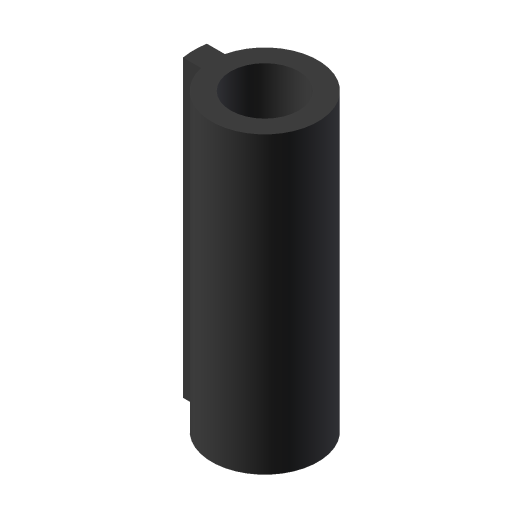
# Autodesk Inventor part: Servo Adapter
Saved by Autodesk Inventor 2023.4 (Build 274418000, 418)
## iProperties
Created: 2024-02-27
Part Number: Servo Adapter
Material: Generic
Document SubType Name: Modeling
Designer: josep
Density: 1 g/cm^3
Appearance: Default
Author: josep
Autodesk Inventor part; units mm, degrees
ref_plane "YZ Plane" through (0, 0, 0) normal (1, 0, 0) x (0, 1, 0)
ref_plane "XZ Plane" through (0, 0, 0) normal (0, 1, 0) x (-1, 0, 0)
ref_plane "XY Plane" through (0, 0, 0) normal (0, 0, 1) x (1, 0, 0)
sketch "Sketch1" plane through (0, 0, 0) normal (0, 1, 0) x (-1, 0, 0)
  circle A0 centre (0, 0) radius 4.5
  circle A1 centre (0, 0) radius 2.9
  circle A2 centre (0, 0) radius 6
  line L0 (4.3875, -1) -> (5.9161, -1)
  line L1 (4.3875, 1) -> (5.9161, 1)
  dimension "d0" = 0
  dimension "d1" = 0
  dimension "d2" = 9
  dimension "d3" = 5.8
  dimension "d4" = 12
  dimension "d5" = 1
  dimension "d6" = 1
  constraints: 4 end point, 4 point on circle, 3 centre point, 2 coincident, 1 horizontal, 1 parallel
  measures "d0" distance of point (0, 0) A0.centre
  measures "d1" distance of point (0, 0) A0.centre
  measures "d2" diameter of A0
  measures "d3" diameter of A1
  measures "d4" diameter of A2
  measures "d5" vertical distance of A1.centre L1.start
  measures "d6" vertical distance of A1.centre L0.end
extrude "Extrusion1" add sketch "Sketch1" along normal blind 25 contours A0 | A0 L1 A2 L0 picked at (4.9667, 0.558)
body "Solid1"
